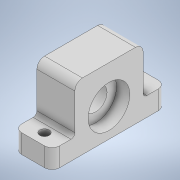
# Autodesk Inventor part: Soporte_rueda_aluminio
Saved by Autodesk Inventor 2022 (Build 260153000, 153)
## iProperties
Created: 2022-12-06
Part Number: Soporte_rueda_aluminio
Material: Genérico
Document SubType Name: Modeling
Designer: Usuario
Density: 1 g/cm^3
Appearance: Valor por defecto
Author: Usuario
Autodesk Inventor part; units mm, degrees
ref_plane "YZ Plane" through (0, 0, 0) normal (1, 0, 0) x (0, 1, 0)
ref_plane "XZ Plane" through (0, 0, 0) normal (0, 1, 0) x (-1, 0, 0)
ref_plane "XY Plane" through (0, 0, 0) normal (0, 0, 1) x (1, 0, 0)
sketch "Boceto1" plane through (0, 0, 0) normal (1, 0, 0) x (0, 1, 0)
  line L0 (0, 0) -> (0, -60)
  line L1 (0, -60) -> (10, -60)
  line L2 (10, -60) -> (10, -48)
  line L3 (10, -48) -> (35, -48)
  line L4 (35, -48) -> (35, -12)
  line L5 (35, -12) -> (10, -12)
  line L6 (10, -12) -> (10, 0)
  line L7 (10, 0) -> (0, 0)
  circle A0 centre (15, -30) radius 6
  dimension "d0" = 36
  dimension "d1" = 12
  dimension "d2" = 12
  dimension "d3" = 35
  dimension "d4" = 10
  dimension "d5" = 20
  dimension "d6" = 18
  dimension "d7" = 12
  constraints: 16 end point, 6 perpendicular, 2 point on line, 1 centre point, 1 vertical
  measures "d0" distance between parallel lines of L3 L5
  measures "d1" distance between parallel lines of L5 L7
  measures "d2" distance between parallel lines of L1 L3
  measures "d3" distance between parallel lines of L4 L0
  measures "d4" distance between parallel lines of L6 L0
  measures "d5" distance from line of A0.centre L4
  measures "d6" distance from line of A0.centre L5
  measures "d7" diameter of A0
extrude "Extrusión1" add sketch "Boceto1" along normal blind 20
sketch "Boceto2" plane through (20, 0, 0) normal (1, 0, 0) x (0, 0, -1)
  circle A0 centre (30, 15) radius 6 projected
  circle A1 centre (30, 15) radius 11
  point P0 (0, 0)
  dimension "d10" = 22
  constraints: 1 centre point, 1 coincident
  measures "d10" diameter of A1
extrude "Extrusión2" cut sketch "Boceto2" against normal blind 7
sketch "Boceto3" plane through (0, 0, 0) normal (-1, 0, 0) x (0, 0, 1)
  circle A0 centre (-30, 15) radius 6 projected
  circle A1 centre (-30, 15) radius 11
  point P0 (0, 0)
  dimension "d13" = 22
  constraints: 1 centre point, 1 coincident
  measures "d13" diameter of A1
extrude "Extrusión3" cut sketch "Boceto3" against normal blind 7
sketch "Boceto4" plane through (0, 10, 0) normal (0, 1, 0) x (1, 0, 0)
  line L0 (20, 12) -> (20, 0) projected
  line L1 (0, 12) -> (0, 0) projected
  line L2 (20, 60) -> (20, 48) projected
  line L3 (0, 12) -> (20, 12) projected
  line L4 (0, 0) -> (20, 0) projected
  line L5 (0, 60) -> (20, 60) projected
  point P0 (10, 6)
  point P1 (10, 54.3165)
  dimension "d16" = 20
  dimension "d17" = 10
  dimension "d18" = 10
  dimension "d19" = 12
  dimension "d20" = 6
  dimension "d21" = 5.6836
  measures "d16" distance between parallel lines of L0 L1
  measures "d17" distance from line of point (10, 6) L0
  measures "d18" distance from line of point (10, 54.316) L2
  measures "d19" distance between parallel lines of L3 L4
  measures "d20" distance from line of point (10, 6) L4
  measures "d21" distance from line of point (10, 54.316) L5
hole "Agujero1" at (10, 10, -6) at (10, 10, -54.3165) direction (0, -1, 0) diameter 5 end through all
fillet "Empalme1" radius 4 4 edges at (20, 5, 0) (20, 5, -60) (0, 5, -60) (0, 5, 0)
fillet "Empalme2" radius 2 2 edges at (10, 10, -12) (10, 10, -48)
fillet "Empalme3" radius 4 2 edges at (10, 35, -12) (10, 35, -48)
equation "\"d2\" = d1"
equation "\"d6\" = 0.5 * d0"
equation "\"d17\" = 0.5 * d16"
equation "\"d18\" = d17"
equation "\"d20\" = 0.5 * d19"
